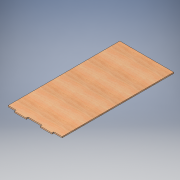
# Autodesk Inventor part: Bottom
Saved by Autodesk Inventor 2016 (Build 200138000, 138)
## iProperties
Created: 2016-02-10
Part Number: Bottom
Material: Wood (Birch)
Document SubType Name: Modeling
Designer: ron
Density: 0.55 g/cm^3
Appearance: Birch - Natural Polished
Mass: 4973.17 g
Surface Area: 14705.4 cm^2
Volume: 9042.13 cm^3
Author: ron
Autodesk Inventor part; units mm, degrees
ref_plane "YZ Plane" through (0, 0, 0) normal (1, 0, 0) x (0, 1, 0)
ref_plane "XZ Plane" through (0, 0, 0) normal (0, 1, 0) x (-1, 0, 0)
ref_plane "XY Plane" through (0, 0, 0) normal (0, 0, 1) x (1, 0, 0)
sketch "Sketch1" plane through (0, 0, 0) normal (0, 1, 0) x (-1, 0, 0)
  line L0 (584.6064, 0) -> (584.6064, -1209.1924)
  line L1 (584.6064, -1209.1924) -> (0, -1209.1924)
  line L2 (0, -1209.1924) -> (0, 0)
  line L3 (584.6064, 0) -> (495.7064, 0)
  line L4 (495.7064, 0) -> (495.7064, 19.9898)
  line L5 (495.7064, 19.9898) -> (368.7064, 19.9898)
  line L6 (368.7064, 19.9898) -> (368.7064, 0)
  line L7 (368.7064, 0) -> (216.3064, 0)
  line L8 (216.3064, 0) -> (216.3064, 19.9898)
  line L9 (216.3064, 19.9898) -> (89.3064, 19.9898)
  line L10 (89.3064, 19.9898) -> (89.3064, 0)
  line L11 (495.7064, 0) -> (584.6064, 0)
  line L12 (0, 0) -> (89.3064, 0)
  line L13 (216.3064, 0) -> (368.7064, 0)
  dimension "d0" = 1209.1924
  dimension "d1" = 584.6064
  dimension "d4" = 88.9
  dimension "d5" = 19.9898
  dimension "d6" = 127
  dimension "d7" = 152.4
  dimension "d8" = 19.9898
  dimension "d9" = 127
  dimension "d10" = 0
  dimension "d11" = 90
  dimension "d12" = 89.3064
  constraints: 28 end point, 11 perpendicular, 4 parallel, 3 horizontal, 2 point on line
  measures "d0" distance of L0.start L0.end
  measures "d1" distance of L0.end L1.end
  measures "d4" distance of L0.start L3.end
  measures "d5" distance of L3.end L4.end
  measures "d6" distance of L4.end L5.end
  measures "d7" distance of L6.end L7.end
  measures "d8" distance of L7.end L8.end
  measures "d9" distance of L8.end L9.end
  measures "d10" distance between parallel lines of L12 L7
  measures "d11" angle of L8 L9
  measures "d12" distance of L2.end L10.end
extrude "Extrusion1" add sketch "Sketch1" along normal blind 12.7
body "Solid1"
